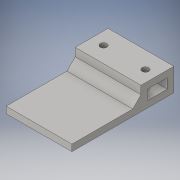
# Autodesk Inventor part: Hotend holder V4 Beltmount
Saved by Autodesk Inventor 2016 (Build 200138000, 138)
## iProperties
Created: 2016-02-19
Part Number: Hotend holder V4 Beltmount
Material: Generic
Document SubType Name: Modeling
Designer: Scott
Density: 1 g/cm^3
Appearance: Default
Author: Scott
Autodesk Inventor part; units mm, degrees
ref_plane "YZ Plane" through (0, 0, 0) normal (1, 0, 0) x (0, 1, 0)
ref_plane "XZ Plane" through (0, 0, 0) normal (0, 1, 0) x (-1, 0, 0)
ref_plane "XY Plane" through (0, 0, 0) normal (0, 0, 1) x (1, 0, 0)
sketch "Sketch1" plane through (0, 0, 0) normal (0, 1, 0) x (-1, 0, 0)
  line L0 (0, 0) -> (25.4, 0)
  line L1 (25.4, 0) -> (25.4, -25.4)
  line L2 (25.4, -25.4) -> (0, -25.4)
  line L3 (0, -25.4) -> (0, 0)
  dimension "d0" = 25.4
  dimension "d1" = 25.4
  constraints: 8 end point, 2 parallel, 1 horizontal, 1 perpendicular
  measures "d0" distance of L1.end L2.end
  measures "d1" distance of L0.end L1.end
extrude "Extrusion1" add sketch "Sketch1" along normal blind 2.54
sketch "Sketch2" plane through (0, 2.54, 0) normal (0, 1, 0) x (1, 0, 0)
  line L0 (0, 25.4) -> (-25.4, 25.4) projected
  line L1 (-25.4, 25.4) -> (0, 25.4)
  line L2 (0, 25.4) -> (0, 24.13)
  line L3 (0, 24.13) -> (-25.4, 24.13)
  line L4 (-25.4, 24.13) -> (-25.4, 25.4)
  line L5 (-12.7, 24.13) -> (-12.7, 16.51)
  line L6 (-12.7, 24.13) -> (-5.08, 24.13) construction
  line L7 (-25.4, 16.51) -> (0, 16.51)
  line L8 (0, 16.51) -> (0, 13.97)
  line L9 (0, 13.97) -> (-25.4, 13.97)
  line L10 (-25.4, 13.97) -> (-25.4, 16.51)
  point P0 (0, 0)
  dimension "d4" = 25.4
  dimension "d5" = 1.27
  dimension "d6" = 7.62
  dimension "d7" = 90
  dimension "d8" = 25.4
  dimension "d9" = 2.54
  constraints: 20 end point, 4 parallel, 3 horizontal, 3 perpendicular, 1 midpoint, 1 vertical
  measures "d4" distance of L2.end L3.end
  measures "d5" distance of L1.end L2.end
  measures "d6" distance of L5.start L5.end
  measures "d7" angle of L5 L6
  measures "d8" distance of L8.end L9.end
  measures "d9" distance of L7.end L8.end
extrude "Extrusion2" add sketch "Sketch2" along normal blind 3.81
sketch "Sketch3" plane through (0, 6.35, 0) normal (0, 1, 0) x (1, 0, 0)
  line L0 (0, 13.97) -> (0, 16.51) projected
  line L1 (-25.4, 25.4) -> (0, 25.4) projected
  line L2 (0, 13.97) -> (-25.4, 13.97)
  line L3 (-25.4, 13.97) -> (-25.4, 25.4)
  line L4 (-25.4, 25.4) -> (0, 25.4)
  line L5 (0, 25.4) -> (0, 13.97)
  point P0 (0, 0)
  constraints: 8 end point, 2 parallel, 1 horizontal, 1 perpendicular
extrude "Extrusion3" add sketch "Sketch3" along normal blind 2.54
chamfer "Chamfer1" distance 3.175 angle 45 1 edges at (-12.7, 2.54, -13.97)
sketch "Sketch4" plane through (0, 8.89, 0) normal (0, 1, 0) x (1, 0, 0)
  circle A0 centre (-20.546, 20.0791) radius 1.27
  circle A1 centre (-4.3777, 20.0791) radius 1.27
  point P0 (0, 0)
  dimension "d17" = 2.54
  dimension "d18" = 2.54
  constraints: 2 centre point
  measures "d17" diameter of A0
  measures "d18" diameter of A1
extrude "Extrusion4" cut sketch "Sketch4" against normal blind 25.4
sketch "Sketch5" plane through (-25.4, 0, 0) normal (0, 0, 1) x (1, 0, 0)
  line L0 (0, 2.54) -> (25.4, 2.54) projected
  line L1 (25.4, 0) -> (0, 0) projected
  line L2 (0, 2.54) -> (25.4, 2.54)
  line L3 (25.4, 2.54) -> (25.4, 0)
  line L4 (25.4, 0) -> (0, 0)
  line L5 (0, 0) -> (0, 2.54)
  constraints: 8 end point, 2 parallel, 1 horizontal, 1 perpendicular
extrude "Extrusion5" add sketch "Sketch5" along normal blind 12.7
sketch "Sketch6" plane through (0, 0, -25.4) normal (0, 0, -1) x (-1, 0, 0)
  line L0 (25.4, 0) -> (0, 0) projected
  line L1 (25.4, 0) -> (25.4, 8.89) projected
  line L2 (0, 8.89) -> (25.4, 8.89) projected
  line L3 (0, 0) -> (0, 8.89) projected
extrude "Extrusion6" add sketch "Sketch6" along normal blind 1.27
body "Solid1"
